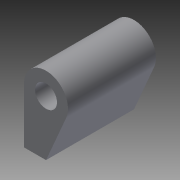
# Autodesk Inventor part: Servo Mount
Saved by Autodesk Inventor 2014 SP1 (Build 180222100, 222)
## iProperties
Created: 2014-01-26
Part Number: Servo Mount
Material: Generic
Document SubType Name: Modeling
Designer: tom
Density: 1 g/cm^3
Appearance: Default
Author: tom
Autodesk Inventor part; units mm, degrees
ref_plane "YZ Plane" through (0, 0, 0) normal (1, 0, 0) x (0, 1, 0)
ref_plane "XZ Plane" through (0, 0, 0) normal (0, 1, 0) x (-1, 0, 0)
ref_plane "XY Plane" through (0, 0, 0) normal (0, 0, 1) x (1, 0, 0)
sketch "Sketch1" plane through (0, 0, 0) normal (0, 0, 1) x (1, 0, 0)
  circle A0 centre (0, 0) radius 3.175
  circle A1 centre (0, 0) radius 6.35
  line L0 (0, -16) -> (5.8285, -2.5202)
  line L1 (0, -16) -> (-6.35, -16)
  line L2 (-6.35, -16) -> (-6.35, 0)
  dimension "d0" = 6.35
  dimension "d1" = 12.7
  constraints: 6 end point, 2 centre point, 2 coincident, 2 point on circle, 2 tangent
  measures "d0" diameter of A0
  measures "d1" diameter of A1
extrude "Extrusion1" add sketch "Sketch1" against normal blind 25.4
sketch "Sketch6" plane through (0, 0, -25.4) normal (0, 0, -1) x (-1, 0, 0)
  line L0 (-5.8285, -2.5202) -> (0, -16) projected
  line L1 (0, -16) -> (6.35, -16) projected
  line L2 (6.35, -16) -> (6.35, 0) projected
  arc A0 (6.35, 0) -> (-5.8285, -2.5202) centre (0, 0) ccw projected
  circle A1 centre (0, 0) radius 6.35
  constraints: 1 centre point, 1 coincident, 1 concentric
extrude "Extrusion5" cut sketch "Sketch6" against normal blind 10 contours A1 L2 L1 L0
body "Solid1"
